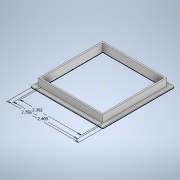
# Autodesk Inventor part: VRSPAD-144 illumination base
Saved by Autodesk Inventor 2022 (Build 260153000, 153)
## iProperties
Created: 2023-04-04
Part Number: VRSPAD-144 illumination base
Material: Generic
Document SubType Name: Modeling
Designer: William
Density: 1 g/cm^3
Appearance: Default
Author: William
Autodesk Inventor part; units mm, degrees
ref_plane "YZ Plane" through (0, 0, 0) normal (1, 0, 0) x (0, 1, 0)
ref_plane "XZ Plane" through (0, 0, 0) normal (0, 1, 0) x (-1, 0, 0)
ref_plane "XY Plane" through (0, 0, 0) normal (0, 0, 1) x (1, 0, 0)
sketch "Sketch1" plane through (0, 0, 0) normal (0, 1, 0) x (-1, 0, 0)
  line L0 (-30, 30) -> (30, 30)
  line L1 (30, 30) -> (30, -30)
  line L2 (30, -30) -> (-30, -30)
  line L3 (-30, -30) -> (-30, 30)
  line L4 (-31.35, 31.35) -> (31.35, 31.35)
  line L5 (31.35, 31.35) -> (31.35, -31.35)
  line L6 (31.35, -31.35) -> (-31.35, -31.35)
  line L7 (-31.35, -31.35) -> (-31.35, 31.35)
  line L8 (-35, 35) -> (35, 35)
  line L9 (35, 35) -> (35, -35)
  line L10 (35, -35) -> (-35, -35)
  line L11 (-35, -35) -> (-35, 35)
  point P0 (0, 0)
  point P1 (0, -30)
  point P2 (0, -31.35)
  point P3 (0, -35)
  point P4 (30, 0)
  point P5 (31.35, 0)
  point P6 (35, 0)
  dimension "d0" = 60
  dimension "d1" = 62.7
  dimension "d2" = 70
  constraints: 24 end point, 6 midpoint, 6 parallel, 6 perpendicular, 3 horizontal, 3 horizontal alignment, 3 vertical alignment
  measures "d0" distance of L0.start L0.end
  measures "d1" distance of L4.start L4.end
  measures "d2" distance of L8.start L8.end
extrude "Extrusion1" add sketch "Sketch1" along normal blind 8 contours L4 L5 L6 L7
extrude "Extrusion2" add sketch "Sketch1" along normal blind 1 contours L8 L9 L10 L11
body "Solid1"
